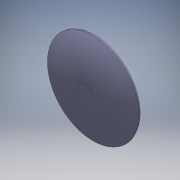
# Autodesk Inventor part: 240516_cup2
Saved by Autodesk Inventor 2016 (Build 200138000, 138)
## iProperties
Created: 2024-05-16
Part Number: 240516_cup2
Material: 일반
Document SubType Name: Modeling
Designer: pc
Density: 1 g/cm^3
Appearance: 슬레이트 파란색
Author: pc
Autodesk Inventor part; units mm, degrees
ref_plane "YZ Plane" through (0, 0, 0) normal (1, 0, 0) x (0, 1, 0)
ref_plane "XZ Plane" through (0, 0, 0) normal (0, 1, 0) x (-1, 0, 0)
ref_plane "XY Plane" through (0, 0, 0) normal (0, 0, 1) x (1, 0, 0)
sketch "스케치1" plane through (0, 0, 0) normal (0, 0, 1) x (1, 0, 0)
  line L0 (0, 3.6283) -> (8, 3.6283)
  arc A0 (-42.6971, 12.9288) -> (0, 3.6283) centre (-2.6602, 94.0741) ccw
  arc A1 (-43.9855, 10.4041) -> (0.0413, 0.7941) centre (-2.6602, 94.0741) ccw
  line L1 (0.0413, 0.7941) -> (8, 0.7941)
  line L2 (-43.9855, 10.4041) -> (-42.6971, 12.9288)
  line L3 (8, 0.7941) -> (8, 3.6283)
  point P0 (0, 0)
  dimension "d0" = 8
  constraints: 8 end point, 4 point on circle, 2 centre point, 1 horizontal, 1 vertical, 1 other
  measures "d0" distance of L0.start L0.end
revolve "회전1" add sketch "스케치1" angle 360 about axis through (8, 0.7941, 0) along (0, 1, 0)
fillet "모깎기1" radius 0.5 2 edges at (58.6971, 12.9288, 0) (59.9855, 10.4041, 0)
